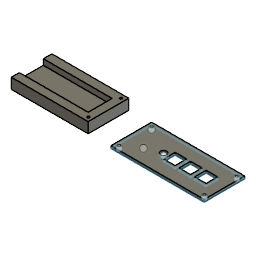
Hippogriff's Hack Pad (Autodesk Fusion 360 design; units mm, degrees)
part number: 2026-03-31-14-26-59-995
Autodesk Fusion 360 part; units mm, degrees
sketch "Sketch1" plane through (0, 0, 0) normal (0, 1, 0) x (1, 0, 0)
  line L0 (-9.7865, 19.4) -> (84.6135, 19.4)
  line L1 (84.6135, 19.4) -> (84.6135, -10)
  line L2 (84.6135, -10) -> (-9.7865, -10)
  line L3 (-9.7865, -10) -> (-9.7865, 19.4)
  line L4 (-20, 30) -> (94.6135, 30)
  line L5 (94.6135, 30) -> (94.6135, -20)
  line L6 (94.6135, -20) -> (-20, -20)
  line L7 (-20, -20) -> (-20, 30)
  circle A0 centre (-15, 25) radius 1.45
  circle A1 centre (-15, -15) radius 1.45
  circle A2 centre (90, -15) radius 1.45
  circle A3 centre (90, 25) radius 1.45
  dimension "d1" = 94.4
  dimension "d2" = 29.4
  dimension "d5" = 2.9
  dimension "d6" = 2.9
  dimension "d7" = 2.9
  dimension "d8" = 2.9
  constraint horizontal L0
  constraint vertical L1
  constraint horizontal L2
  constraint vertical L3
  constraint horizontal L4
  constraint vertical L5
  constraint horizontal L6
  constraint vertical L7
  measures "d1" distance of L0.start L0.end
  measures "d2" distance of L0.end L1.end
  measures "d5" diameter of A0
  measures "d6" diameter of A1
  measures "d7" diameter of A2
  measures "d8" diameter of A3
extrude "Extrude4" add sketch "Sketch1" along normal blind 13 makes body 1
extrude "Extrude5" add sketch "Sketch1" along normal blind 3 contours L0 L1 L2 L3 bodies 1
sketch "kbplate" plane through (0, 0, 0) normal (0, 1, 0) x (1, 0, 0)
  line L0 (170.778, -3.2441) -> (184.778, -3.2441)
  line L1 (184.778, 10.7559) -> (170.778, 10.7559)
  line L2 (184.778, -3.2441) -> (184.778, 10.7559)
  line L3 (170.778, 10.7559) -> (170.778, -3.2441)
  line L4 (189.828, -3.2441) -> (203.828, -3.2441)
  line L5 (203.828, 10.7559) -> (189.828, 10.7559)
  line L6 (203.828, -3.2441) -> (203.828, 10.7559)
  line L7 (189.828, 10.7559) -> (189.828, -3.2441)
  line L8 (208.878, -3.2441) -> (222.878, -3.2441)
  line L9 (222.878, 10.7559) -> (208.878, 10.7559)
  line L10 (222.878, -3.2441) -> (222.878, 10.7559)
  line L11 (208.878, 10.7559) -> (208.878, -3.2441)
  circle A0 centre (164.2894, 3.1324) radius 3.75
  circle A1 centre (129.135, -16.5252) radius 1.45
  line L12 (238.7484, -21.5252) -> (124.135, -21.5252)
  line L13 (124.135, 28.4748) -> (238.7484, 28.4748)
  circle A2 centre (234.135, 23.4748) radius 1.45
  circle A3 centre (234.135, -16.5252) radius 1.45
  circle A4 centre (129.135, 23.4748) radius 1.45
  line L14 (238.7484, 28.4748) -> (238.7484, -21.5252)
  line L15 (124.135, -21.5252) -> (124.135, 28.4748)
  point P0 (144.135, -1.5252)
  dimension "d21" = 7.5
  dimension "d30" = 2.9
  dimension "d31" = 2.9
  dimension "d32" = 2.9
  dimension "d33" = 2.9
  constraint horizontal L13
  constraint vertical L14
  constraint horizontal L12
  constraint vertical L15
  measures "d21" diameter of A0
  measures "d30" diameter of A4
  measures "d31" diameter of A1
  measures "d32" diameter of A3
  measures "d33" diameter of A2
extrude "Extrude6" add 1 faces at (53.1468, 3, 0.2) along direction (0, 1, 0) blind 3 on bodies 1 bodies 1
extrude "Extrude9" add sketch "kbplate" along normal blind 3 separate body makes body 2
extrude "Extrude10" cut 1 faces at (-20, 4.3333, 3.3333) along direction (1, 0, 0) blind 10 on bodies 1 bodies 1
extrude "Extrude11" cut 1 faces at (-10, 4.3333, 3.3333) along direction (1, 0, 0) blind 10 on bodies 1 bodies 1
sketch "Sketch6" plane through (0, 0, 0) normal (1, 0, 0) x (0, 0, -1)
